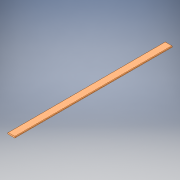
# Autodesk Inventor part: Kertdeszka
Saved by Autodesk Inventor 2019 (Build 230136000, 136)
## iProperties
Created: 2025-01-08
Part Number: Kertdeszka
Material: Wood (Cherry)
Document SubType Name: Modeling
Designer: laca
Density: 0.63 g/cm^3
Appearance: Cherry - Natural Low Gloss
Mass: 6511.17 g
Surface Area: 9556.87 cm^2
Volume: 10335.2 cm^3
m3 beton: 0.0
Author: laca
Autodesk Inventor part; units mm, degrees
ref_plane "YZ Plane" through (0, 0, 0) normal (1, 0, 0) x (0, 1, 0)
ref_plane "XZ Plane" through (0, 0, 0) normal (0, 1, 0) x (-1, 0, 0)
ref_plane "XY Plane" through (0, 0, 0) normal (0, 0, 1) x (1, 0, 0)
sketch "Sketch1" plane through (0, 0, 0) normal (0, 0, 1) x (1, 0, 0)
  line L0 (0, 0) -> (-140, 0)
  line L1 (-140, 0) -> (-140, 28)
  line L2 (-140, 28) -> (0, 28)
  line L3 (0, 28) -> (0, 0)
  dimension "d0" = 140
  dimension "d1" = 28
  constraints: 8 end point, 2 parallel, 1 horizontal, 1 perpendicular
  measures "d0" distance of L1.end L2.end
  measures "d1" distance of L0.end L1.end
extrude "Extrusion1" add sketch "Sketch1" along normal blind 3000
fillet "Fillet1" radius 8 4 edges at (0, 28, 1500) (0, 0, 1500) (-140, 28, 1500) (-140, 0, 1500)
body "Solid1"
